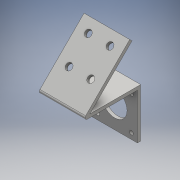
# Autodesk Inventor part: 电机座1
Saved by Autodesk Inventor 2016 (Build 200138000, 138)
## iProperties
Created: 2019-04-02
Part Number: 电机座1
Material: 常规
Document SubType Name: Modeling
Designer: oldboy
Density: 1 g/cm^3
Appearance: 默认
Author: oldboy
Autodesk Inventor part; units mm, degrees
ref_plane "YZ Plane" through (0, 0, 0) normal (1, 0, 0) x (0, 1, 0)
ref_plane "XZ Plane" through (0, 0, 0) normal (0, 1, 0) x (-1, 0, 0)
ref_plane "XY Plane" through (0, 0, 0) normal (0, 0, 1) x (1, 0, 0)
sketch "草图2" plane through (0, 0, 0) normal (0, 1, 0) x (-1, 0, 0)
  line L0 (-21, 21) -> (21, 21)
  line L1 (21, 21) -> (21, -21)
  line L2 (21, -21) -> (-21, -21)
  line L3 (-21, -21) -> (-21, 21)
  line L4 (-21, 21) -> (21, -21) construction
  line L5 (21, 21) -> (-21, -21) construction
  point P0 (0, 0)
  dimension "d3" = 42
  dimension "d4" = 42
  constraints: 12 end point, 2 midpoint, 2 parallel, 1 horizontal, 1 perpendicular
  measures "d3" distance between parallel lines of L3 L1
  measures "d4" distance between parallel lines of L2 L0
extrude "拉伸2" add sketch "草图2" along normal blind 3
sketch "草图3" plane through (-21, 0, 21) normal (0, 0, 1) x (1, 0, 0)
  line L0 (0, 3) -> (42, 3) projected
  line L1 (0, 3) -> (42, 3)
  line L2 (42, 3) -> (42, -48)
  line L3 (42, -48) -> (0, -48)
  line L4 (0, -48) -> (0, 3)
  point P0 (21, 0)
  dimension "d7" = 51
  constraints: 8 end point, 2 parallel, 1 horizontal, 1 perpendicular
  measures "d7" distance between parallel lines of L3 L0
extrude "拉伸3" add sketch "草图3" along normal blind 3
ref_plane "工作平面1" through (-21, -48, 24) normal (0, -0.7071068, 0.7071068) x (1, 0, 0)
sketch "草图4" plane through (-21, -48, 24) normal (0, -0.7071068, 0.7071068) x (1, 0, 0)
  line L0 (0, -2.1213) -> (42, -2.1213) projected
  line L1 (0, 31.8198) -> (0, -2.1213) projected
  line L2 (0, 0) -> (0, 57.8787)
  line L3 (0, 57.8787) -> (42, 57.8787)
  line L4 (42, 57.8787) -> (42, 0)
  line L5 (0, 0) -> (42, 0) projected
  point P0 (21, 16.9706)
  dimension "d11" = 60
  constraints: 6 end point, 2 point on line, 1 parallel
  measures "d11" distance between parallel lines of L3 L0
extrude "拉伸4" add sketch "草图4" against normal blind 3
sketch "草图6" plane through (-21, 0, -21) normal (-1, 0, 0) x (0, 0, 1)
  line L0 (42, 0) -> (42, -48) construction
  line L1 (104.9558, 11.9558) -> (7.0074, -85.9926) construction
  line L2 (42, -48) -> (42, -51)
  line L3 (42, -48) -> (45, -48) projected
  line L4 (42, -51) -> (45, -48)
  line L5 (45, -48) -> (42, -48)
  point P0 (21, 0)
  constraints: 6 end point, 1 collinear, 1 point on line, 1 vertical
extrude "拉伸5" add sketch "草图6" against normal up to surface (42 mm away)
fillet "圆角1" radius 2 1 edges at (0, -51, 21)
sketch "草图7" plane through (0, 0, 0) normal (0, -1, 0) x (1, 0, 0)
  circle A0 centre (0, 0) radius 11.5
  circle A1 centre (-15.5, 15.5) radius 1.75
  circle A2 centre (-15.5, -15.5) radius 1.75
  circle A3 centre (15.5, -15.5) radius 1.75
  circle A4 centre (15.5, 15.5) radius 1.75
  dimension "d17" = 23
  dimension "d18" = 3.5
  dimension "d19" = 15.5
  dimension "d20" = 15.5
  dimension "d21" = 15.5
  dimension "d22" = 15.5
  constraints: 5 centre point, 3 equal radius, 2 horizontal alignment, 2 vertical alignment, 1 coincident
  measures "d17" diameter of A0
  measures "d18" diameter of A2
  measures "d19" horizontal distance of point (0, 0) A2.centre
  measures "d20" horizontal distance of point (0, 0) A2.centre
  measures "d21" horizontal distance of point (0, 0) A1.centre
  measures "d22" horizontal distance of point (0, 0) A3.centre
extrude "拉伸6" cut sketch "草图7" against normal blind 3
sketch "草图8" plane through (-21, -48, 24) normal (0, -0.7071068, 0.7071068) x (1, 0, 0)
  line L0 (0, 57.8787) -> (42, 57.8787) projected
  line L1 (21, 57.8787) -> (21, 0.5858) construction
  line L2 (42, 0.5858) -> (0, 0.5858) projected
  circle A0 centre (31, 22.8787) radius 3
  circle A1 centre (31, 47.8787) radius 3
  circle A2 centre (11, 22.8787) radius 3
  circle A3 centre (11, 47.8787) radius 3
  point P0 (21, 16.9706)
  dimension "d25" = 6
  dimension "d26" = 6
  dimension "d27" = 10
  dimension "d28" = 25
  dimension "d29" = 10
  constraints: 4 centre point, 2 end point, 2 midpoint, 2 symmetric about line, 1 vertical alignment, 2 other
  measures "d25" diameter of A0
  measures "d26" diameter of A1
  measures "d27" distance from line of L1 A0.centre
  measures "d28" distance of A1.centre A0.centre
  measures "d29" distance from line of L0 A1.centre
extrude "拉伸7" cut sketch "草图8" against normal blind 3
